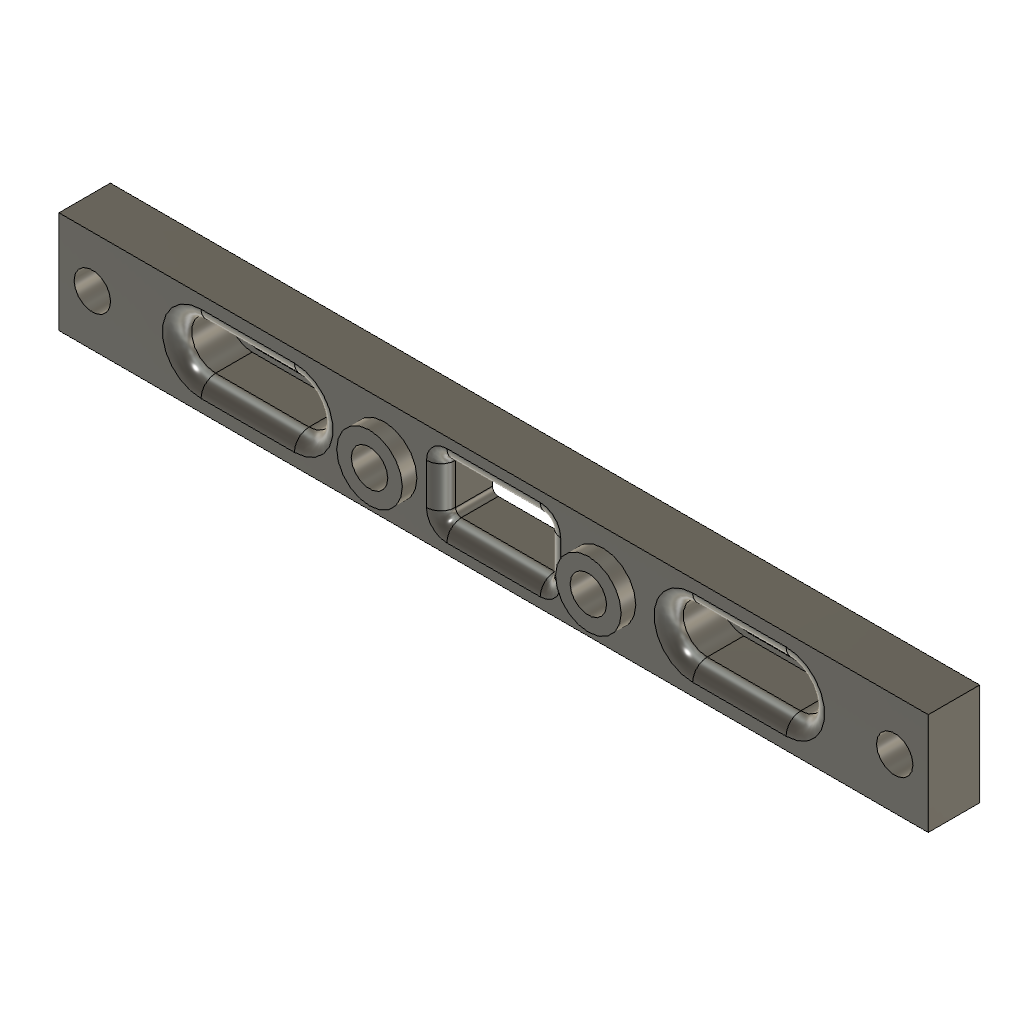
USB SW Plate (Autodesk Fusion 360 design; units mm, degrees)
Autodesk Fusion 360 part; units mm, degrees
note: some values were not read from the file. Set by a fixed rule: which sketch regions a step uses.
sketch "Sketch1" plane through (0, 0, 0) normal (0, 1, 0) x (1, 0, 0)
  line L0 (0, 0) -> (60, 0)
  line L1 (60, 0) -> (60, -7)
  line L2 (60, -7) -> (0, -7)
  line L3 (0, -7) -> (0, 0)
  line L4 (0, -7) -> (2.5, -7)
  line L5 (2.5, -7) -> (2.5, -3.5)
  line L6 (2.5, -3.5) -> (0, -3.5)
  line L7 (0, -3.5) -> (0, -7)
  line L8 (60, -7) -> (57.5, -7)
  line L9 (57.5, -7) -> (57.5, -3.5)
  line L10 (57.5, -3.5) -> (60, -3.5)
  line L11 (60, -3.5) -> (60, -7)
  circle A0 centre (2.5, -3.5) radius 1.25
  circle A1 centre (57.5, -3.5) radius 1.25
  line L12 (0, -7) -> (30, -7)
  line L13 (30, -7) -> (30, -3.5)
  line L14 (30, -3.5) -> (26.4, -3.5)
  line L15 (26.4, -3.5) -> (26.4, -5.3)
  line L16 (26.4, -5.3) -> (33.6, -5.3)
  line L17 (33.6, -5.3) -> (33.6, -1.7)
  line L18 (33.6, -1.7) -> (26.4, -1.7)
  line L19 (26.4, -1.7) -> (26.4, -5.3)
  line L20 (30, -3.5) -> (22.5, -3.5)
  line L21 (30, -3.5) -> (37.5, -3.5)
  circle A2 centre (22.5, -3.5) radius 1.25
  circle A3 centre (37.5, -3.5) radius 1.25
  line L22 (30, -3.5) -> (30, -0.5)
  line L23 (30, -0.5) -> (20, -0.5)
  line L24 (20, -0.5) -> (40, -0.5)
  line L25 (40, -0.5) -> (40, -6.5)
  line L26 (40, -6.5) -> (20, -6.5)
  line L27 (20, -6.5) -> (20, -0.5)
  line L28 (0, -7) -> (18, -7)
  line L29 (18, -7) -> (18, -5.15)
  line L30 (18, -5.15) -> (8.3, -5.15)
  line L31 (8.3, -5.15) -> (8.3, -1.85)
  line L32 (8.3, -1.85) -> (18, -1.85)
  line L33 (18, -1.85) -> (18, -5.15)
  line L34 (60, -7) -> (42, -7)
  line L35 (42, -7) -> (42, -5.15)
  line L36 (42, -5.15) -> (51.7, -5.15)
  line L37 (51.7, -5.15) -> (51.7, -1.85)
  line L38 (51.7, -1.85) -> (42, -1.85)
  line L39 (42, -1.85) -> (42, -5.15)
  line L40 (42, -5.15) -> (42, -4.8)
  line L41 (42, -4.8) -> (42.7, -4.8)
  line L42 (42.7, -4.8) -> (51, -4.8)
  line L43 (51, -4.8) -> (51, -2.2)
  line L44 (51, -2.2) -> (42.7, -2.2)
  line L45 (42.7, -2.2) -> (42.7, -4.8)
  line L46 (18, -5.15) -> (18, -4.8)
  line L47 (18, -4.8) -> (17.3, -4.8)
  line L48 (17.3, -4.8) -> (9, -4.8)
  line L49 (9, -4.8) -> (9, -2.2)
  line L50 (9, -2.2) -> (17.3, -2.2)
  line L51 (17.3, -2.2) -> (17.3, -4.8)
  circle A4 centre (22.5, -3.5) radius 2.25
  circle A5 centre (37.5, -3.5) radius 2.25
  dimension "d1" = 60
  dimension "d2" = 7
  dimension "d3" = 2.5
  dimension "d4" = 3.5
  dimension "d5" = 2.5
  dimension "d6" = 3.5
  dimension "d7" = 2.5
  dimension "d8" = 2.5
  dimension "d11" = 30
  dimension "d12" = 3.5
  dimension "d13" = 3.6
  dimension "d14" = 1.8
  dimension "d15" = 7.2
  dimension "d16" = 3.6
  dimension "d17" = 7.5
  dimension "d18" = 7.5
  dimension "d19" = 2.5
  dimension "d20" = 2.5
  dimension "d21" = 3
  dimension "d22" = 10
  dimension "d23" = 20
  dimension "d24" = 6
  dimension "d25" = 18
  dimension "d26" = 1.85
  dimension "d27" = 9.7
  dimension "d28" = 3.3
  dimension "d29" = 18
  dimension "d30" = 1.85
  dimension "d31" = 9.7
  dimension "d32" = 3.3
  dimension "d33" = 0.7
  dimension "d34" = 8.3
  dimension "d35" = 2.6
  dimension "d36" = 0.35
  dimension "d37" = 0.35
  dimension "d38" = 0.7
  dimension "d39" = 8.3
  dimension "d40" = 2.6
  dimension "d45" = 4.5
  dimension "d46" = 4.5
  constraint horizontal L0
  constraint vertical L1
  constraint horizontal L2
  constraint vertical L3
  constraint coincident L0.start L3.end
  constraint horizontal L4
  constraint vertical L5
  constraint horizontal L6
  constraint vertical L7
  constraint horizontal L8
  constraint vertical L9
  constraint horizontal L10
  constraint vertical L11
  constraint coincident L5.end L6.start
  constraint coincident L9.end L10.start
  constraint perpendicular L7 L12
  constraint perpendicular L2 L13
  constraint perpendicular L13 L14
  constraint perpendicular L14 L15
  constraint horizontal L16
  constraint vertical L17
  constraint horizontal L18
  constraint vertical L19
  constraint perpendicular L13 L20
  constraint perpendicular L17 L21
  constraint coincident L20.end A2.centre
  constraint coincident L21.end A3.centre
  constraint perpendicular L18 L22
  constraint perpendicular L22 L23
  constraint horizontal L24
  constraint vertical L25
  constraint horizontal L26
  constraint vertical L27
  constraint perpendicular L5 L28
  constraint perpendicular L12 L29
  constraint horizontal L30
  constraint vertical L31
  constraint horizontal L32
  constraint vertical L33
  constraint perpendicular L11 L34
  constraint perpendicular L2 L35
  constraint horizontal L36
  constraint vertical L37
  constraint horizontal L38
  constraint vertical L39
  constraint coincident L39 L40.end
  constraint perpendicular L39 L41
  constraint horizontal L42
  constraint vertical L43
  constraint horizontal L44
  constraint vertical L45
  constraint perpendicular L30 L46
  constraint perpendicular L33 L47
  constraint horizontal L48
  constraint vertical L49
  constraint horizontal L50
  constraint vertical L51
  constraint concentric A2 A4
  measures "d1" distance of L0.start L0.end
  measures "d2" distance of L0.start L2.end
  measures "d3" distance of L2.end L4.end
  measures "d4" distance of L2.end L6.end
  measures "d5" distance of L1.end L8.end
  measures "d6" distance of L1.end L10.end
  measures "d7" diameter of A0
  measures "d8" diameter of A1
  measures "d11" distance of L2.end L12.end
  measures "d12" distance of L12.end L13.end
  measures "d13" distance of L13.end L14.end
  measures "d14" distance of L14.end L15.end
  measures "d15" distance of L15.end L16.end
  measures "d16" distance of L15.end L18.end
  measures "d17" distance of L13.end L20.end
  measures "d18" distance of L13.end L21.end
  measures "d19" diameter of A2
  measures "d20" diameter of A3
  measures "d21" distance of L13.end L22.end
  measures "d22" distance of L22.end L23.end
  measures "d23" distance of L23.end L24.end
  measures "d24" distance of L23.end L26.end
  measures "d25" distance of L2.end L28.end
  measures "d26" distance of L28.end L29.end
  measures "d27" distance of L29.end L30.end
  measures "d28" distance of L29.end L32.end
  measures "d29" distance of L1.end L34.end
  measures "d30" distance of L34.end L35.end
  measures "d31" distance of L35.end L36.end
  measures "d32" distance of L35.end L38.end
  measures "d33" distance of L40.end L41.end
  measures "d34" distance of L41.end L42.end
  measures "d35" distance of L41.end L44.end
  measures "d36" distance of L35.end L40.end
  measures "d37" distance of L29.end L46.end
  measures "d38" distance of L46.end L47.end
  measures "d39" distance of L47.end L48.end
  measures "d40" distance of L47.end L50.end
  measures "d45" diameter of A4
  measures "d46" diameter of A5
extrude "Extrude1" add sketch "Sketch1" along normal blind 3.532 contours L0 L1 L2 L3 L5 L6 L9 L10 A0 A1 L12 L28 L34 | L2 L3 L4 L5 L6 L7 A0 L12 L28 | L1 L2 L8 L9 L10 L11 A1 L34 | L5 L6 A0 | L5 L6 A0 | L9 L10 A1 | L9 L10 A1 | L13 L15 L16 L18 L19 L22 L23 L24 L26 L27 | L13 L16 L17 L18 L22 L24 L25 L26 | L13 L14 L15 L16 L19 L20 | L13 L16 L17 L21 | L17 L18 L21 L22 | L14 L18 L19 L20 L22 | A2 | A3 | L30 L31 L32 L33 L46 | L36 L37 L38 L39 L40 | L42 L43 L44 L45 | L48 L49 L50 L51 | A4 | A5
extrude "Extrude2" cut sketch "Sketch1" along normal blind 4 contours L13 L14 L15 L16 L19 L20 | L13 L16 L17 L21 | L17 L18 L21 L22 | L14 L18 L19 L20 L22 | L42 L43 L44 L45 | L48 L49 L50 L51
extrude "Extrude3" cut sketch "Sketch1" along normal blind 3.5 contours L30 L31 L32 L33 L46 | L36 L37 L38 L39 L40
extrude "Extrude11" cut sketch "Sketch1" along normal blind 2 contours L5 L6 A0 | L5 L6 A0 | L9 L10 A1 | L9 L10 A1
extrude "Extrude4" add sketch "Sketch1" against normal blind 1 contours A4 | A5
extrude "Extrude12" cut 2 faces at (22.4155, 0, 3.409) (37.6522, 0, 3.8879) along direction (0, 1, 0) blind 2
fillet "Fillet1" radius 1.3 8 edges at (51, 3.516, 4.8) (51, 3.516, 2.2) (42.7, 3.516, 4.8) (42.7, 3.516, 2.2) (9, 3.516, 2.2) (9, 3.516, 4.8) (17.3, 3.516, 4.8) (17.3, 3.516, 2.2)
fillet "Fillet2" radius 1.65 8 edges at (18, 1.75, 1.85) (18, 1.75, 5.15) (8.3, 1.75, 5.15) (8.3, 1.75, 1.85) (42, 1.75, 1.85) (42, 1.75, 5.15) (51.7, 1.75, 5.15) (51.7, 1.75, 1.85)
extrude "Extrude7" cut 1 faces at (60, 1.1773, 2.3333) along direction (-1, 0, 0) blind 0.2
extrude "Extrude8" cut 1 faces at (0, 1.1773, 4.6667) along direction (1, 0, 0) blind 0.2
fillet "Fillet3" radius 0.4 4 edges at (26.4, 1.766, 5.3) (26.4, 1.766, 1.7) (33.6, 1.766, 5.3) (33.6, 1.766, 1.7)
fillet "Fillet4" radius 1 16 edges at (42, 0, 3.5) (46.85, 0, 5.15) (51.7, 0, 3.5) (46.85, 0, 1.85) (26.5172, 0, 1.8172) (26.4, 0, 3.5) (26.5172, 0, 5.1828) (30, 0, 5.3) (33.4828, 0, 5.1828) (33.6, 0, 3.5) (33.4828, 0, 1.8172) (30, 0, 1.7) (8.3, 0, 3.5) (13.15, 0, 5.15) (18, 0, 3.5) (13.15, 0, 1.85)
